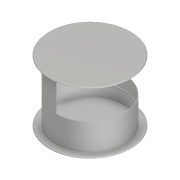
# Autodesk Inventor part: OuterCover
Saved by Autodesk Inventor 2018 (Build 220112000, 112)
## iProperties
Created: 2017-12-09
Part Number: OuterCover
Material: Aluminum 6061
Document SubType Name: Modeling
Designer: Udara Wanasinghe
Density: 2.7 g/cm^3
Appearance: Aluminum - Flat
Mass: 3637.56 g
Surface Area: 8898.74 cm^2
Volume: 1347.25 cm^3
Author: Udara Wanasinghe
Autodesk Inventor part; units mm, degrees
ref_plane "YZ Plane" through (0, 0, 0) normal (1, 0, 0) x (0, 1, 0)
ref_plane "XZ Plane" through (0, 0, 0) normal (0, 1, 0) x (-1, 0, 0)
ref_plane "XY Plane" through (0, 0, 0) normal (0, 0, 1) x (1, 0, 0)
sketch "Sketch1" plane through (0, 0, 0) normal (0, 1, 0) x (-1, 0, 0)
  circle A0 centre (0, 0) radius 158
  circle A1 centre (0, 0) radius 160
  dimension "d0" = 316
  dimension "d1" = 320
  constraints: 2 centre point, 2 coincident
  measures "d0" diameter of A0
  measures "d1" diameter of A1
extrude "Extrusion1" add sketch "Sketch1" along normal blind 240 and the other way blind 40
ref_plane "Work Plane1" through (0, 20, 0) normal (0, -1, 0) x (1, 0, 0)
sketch "Sketch3" plane through (0, 20, 0) normal (0, -1, 0) x (1, 0, 0)
  circle A0 centre (0, 0) radius 158
  circle A1 centre (0, 0) radius 154
  dimension "d8" = 308
  dimension "d16" = 316
  constraints: 2 centre point, 2 coincident
  measures "d8" diameter of A1
  measures "d16" diameter of A0
extrude "Extrusion3" add sketch "Sketch3" against normal blind 4
ref_plane "Work Plane2" through (0, 228, 0) normal (0, 1, 0) x (1, 0, 0)
sketch "Sketch4" plane through (0, 228, 0) normal (0, 1, 0) x (1, 0, 0)
  circle A0 centre (0, 0) radius 158
  circle A1 centre (0, 0) radius 154
  dimension "d12" = 316
  dimension "d13" = 308
  constraints: 2 centre point, 2 coincident
  measures "d12" diameter of A0
  measures "d13" diameter of A1
extrude "Extrusion4" add sketch "Sketch4" along normal blind 4
sketch "Sketch5" plane through (0, 228, 0) normal (0, 1, 0) x (1, 0, 0)
  line L0 (159.9875, -2) -> (-159.9875, -2)
  circle A0 centre (0, 0) radius 160 projected
  arc A1 (-159.9875, -2) -> (159.9875, -2) centre (0, 0) ccw
  dimension "d17" = 2
  constraints: 4 point on circle, 2 end point, 1 centre point, 1 horizontal
  measures "d17" distance from line of L0 point (0, 0)
extrude "Extrusion5" cut sketch "Sketch5" against normal blind 144 contours A0 L0 picked at (22.9687, -49.4673)
sketch "Sketch6" plane through (0, 240, 0) normal (0, 1, 0) x (1, 0, 0)
  circle A0 centre (0, 0) radius 190
  dimension "d22" = 380
  constraints: 1 centre point, 1 coincident
  measures "d22" diameter of A0
extrude "Extrusion6" add sketch "Sketch6" along normal blind 4
fillet "Fillet1" radius 4 1 edges at (-190, 244, 0)
sketch "Sketch7" plane through (0, -40, 0) normal (0, -1, 0) x (1, 0, 0)
  circle A0 centre (0, 0) radius 190
  dimension "d26" = 380
  constraints: 1 centre point, 1 coincident
  measures "d26" diameter of A0
extrude "Extrusion7" add sketch "Sketch7" along normal blind 4
fillet "Fillet2" radius 4 1 edges at (-190, -40, 0)
body "Solid1"
